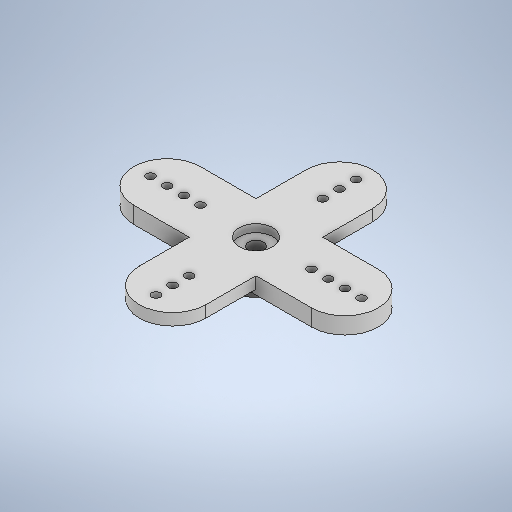
# Autodesk Inventor part: MMAE 232 Assignment 2_Servo Horn 3 - Dylan Tamras
Saved by Autodesk Inventor 2025.2 (Build 292293000, 293)
## iProperties
Created: 2025-01-19
Part Number: MMAE 232 Assignment 2_Servo Horn 3 - Dylan Tamras
Material: Generic
Document SubType Name: Modeling
Designer: Dylan
Density: 1 g/cm^3
Appearance: Default
Author: VRK99-0110
Title: Servo - Horn 3
Autodesk Inventor part; units mm, degrees
ref_plane "YZ Plane" through (0, 0, 0) normal (1, 0, 0) x (0, 1, 0)
ref_plane "XZ Plane" through (0, 0, 0) normal (0, 1, 0) x (-1, 0, 0)
ref_plane "XY Plane" through (0, 0, 0) normal (0, 0, 1) x (1, 0, 0)
sketch "Sketch1" plane through (0, 0, 0) normal (0, 1, 0) x (-1, 0, 0)
  line L0 (6, -15) -> (6, -6)
  line L1 (16, -6) -> (16, 0)
  line L2 (6, -15) -> (0, -15)
  line L3 (16, -6) -> (6, -6)
  arc A0 (0, -21) -> (6, -15) centre (0, -15) ccw
  arc A1 (16, -6) -> (22, 0) centre (16, 0) ccw
  line L4 (6, 15) -> (6, 6)
  line L5 (16, 6) -> (16, 0)
  line L6 (6, 15) -> (0, 15)
  line L7 (16, 6) -> (6, 6)
  arc A2 (6, 15) -> (0, 21) centre (0, 15) ccw
  arc A3 (22, 0) -> (16, 6) centre (16, 0) ccw
  line L8 (-6, -15) -> (-6, -6)
  line L9 (-16, -6) -> (-16, 0)
  line L10 (-6, -15) -> (0, -15)
  line L11 (-16, -6) -> (-6, -6)
  arc A4 (-6, -15) -> (0, -21) centre (0, -15) ccw
  arc A5 (-22, 0) -> (-16, -6) centre (-16, 0) ccw
  line L12 (-16, 6) -> (-16, 0)
  arc A6 (-16, 6) -> (-22, 0) centre (-16, 0) ccw
  line L13 (-16, 6) -> (-6, 6)
  line L14 (-6, 15) -> (-6, 6)
  line L15 (-6, 15) -> (0, 15)
  arc A7 (0, 21) -> (-6, 15) centre (0, 15) ccw
  point P0 (0, 0)
  dimension "d0" = 16
  dimension "d1" = 15
  constraints: 32 end point, 16 point on circle, 8 centre point, 8 coincident, 1 perpendicular, 1 vertical
  measures "d0" distance of point (0, 0) L1.end
  measures "d1" distance of point (0, 0) L2.end
extrude "Extrusion1" add sketch "Sketch1" along normal blind 2.85
sketch "Sketch2" plane through (0, 0, 0) normal (0, -1, 0) x (1, 0, 0)
  line L0 (-6, -15) -> (-6, -6) projected
  line L1 (-6, -6) -> (-6, -15)
  line L2 (6, -6) -> (6, -15) projected
  line L3 (6, -6) -> (6, -15)
  arc A0 (-6, -15) -> (6, -15) centre (0, -15) ccw
  line L4 (-6, -6) -> (6, -6)
  line L5 (-6, 15) -> (-6, 6)
  line L6 (6, 6) -> (6, 15)
  arc A1 (6, 15) -> (-6, 15) centre (0, 15) ccw
  line L7 (-6, 6) -> (6, 6)
  point P0 (0, 0)
  constraints: 12 end point, 4 point on circle, 2 centre point, 2 tangent, 2 vertical
extrude "Extrusion2" cut sketch "Sketch2" against normal blind 1.45
sketch "Sketch3" plane through (0, 2.85, 0) normal (0, 1, 0) x (1, 0, 0)
  circle A0 centre (16, 0) radius 0.75
  circle A1 centre (0, -15) radius 0.75
  circle A2 centre (10, 0) radius 0.75
  circle A3 centre (13, 0) radius 0.75
  circle A4 centre (19, 0) radius 0.75
  arc A5 (6, 15) -> (-6, 15) centre (0, 15) ccw projected
  arc A6 (-6, -15) -> (6, -15) centre (0, -15) ccw projected
  circle A7 centre (-16, 0) radius 0.75
  circle A8 centre (-10, 0) radius 0.75
  circle A9 centre (-13, 0) radius 0.75
  circle A10 centre (-19, 0) radius 0.75
  circle A11 centre (0, -12) radius 0.75
  circle A12 centre (0, -18) radius 0.75
  arc A13 (16, -6) -> (16, 6) centre (16, 0) ccw projected
  arc A14 (-16, 6) -> (-16, -6) centre (-16, 0) ccw projected
  circle A15 centre (0, 15) radius 0.75
  circle A16 centre (0, 12) radius 0.75
  circle A17 centre (0, 18) radius 0.75
  point P0 (0, 0)
  dimension "d10" = 1.5
  dimension "d12" = 1.5
  dimension "d14" = 1.5
  dimension "d17" = 1.5
  dimension "d19" = 1.5
  dimension "d22" = 1.5
  constraints: 14 centre point
  measures "d10" diameter of A1
  measures "d12" diameter of A2
  measures "d14" diameter of A3
  measures "d17" diameter of A4
  measures "d19" diameter of A11
  measures "d22" diameter of A12
extrude "Extrusion3" cut sketch "Sketch3" against normal blind 2.85
sketch "Sketch4" plane through (0, 2.85, 0) normal (0, 1, 0) x (1, 0, 0)
  circle A0 centre (0, 0) radius 3
  dimension "d25" = 6
  constraints: 1 centre point, 1 coincident
  measures "d25" diameter of A0
extrude "Extrusion4" cut sketch "Sketch4" against normal blind 1.4
sketch "Sketch5" plane through (0, 1.45, 0) normal (0, 1, 0) x (1, 0, 0)
  circle A0 centre (0, 0) radius 1.35
  dimension "d28" = 2.7
  constraints: 1 centre point, 1 coincident
  measures "d28" diameter of A0
extrude "Extrusion5" cut sketch "Sketch5" against normal blind 1.45
sketch "Sketch6" plane through (0, 1.45, 0) normal (0, -1, 0) x (1, 0, 0)
  circle A0 centre (0, 18) radius 0.75 projected
  circle A1 centre (0, 12) radius 0.75 projected
  circle A2 centre (0, 15) radius 0.75 projected
  line L0 (6, 6) -> (-6, 6) projected
  line L1 (6, 15) -> (6, 6) projected
  arc A3 (6, 15) -> (-6, 15) centre (0, 15) ccw projected
  line L2 (-6, 6) -> (-6, 15) projected
  point P0 (0, 0)
extrude "Extrusion6" add sketch "Sketch6" along normal blind 0.7
sketch "Sketch7" plane through (0, 1.45, 0) normal (0, -1, 0) x (1, 0, 0)
  circle A0 centre (0, -18) radius 0.75 projected
  circle A1 centre (0, -15) radius 0.75 projected
  circle A2 centre (0, -12) radius 0.75 projected
  line L0 (6, -6) -> (6, -15) projected
  line L1 (-6, -6) -> (6, -6) projected
  line L2 (-6, -15) -> (-6, -6) projected
  arc A3 (-6, -15) -> (6, -15) centre (0, -15) ccw projected
  point P0 (0, 0)
extrude "Extrusion7" add sketch "Sketch7" along normal blind 0.7
sketch "Sketch8" plane through (0, 0, 0) normal (0, -1, 0) x (1, 0, 0)
  circle A0 centre (0, 0) radius 1.35 projected
  circle A1 centre (13, 0) radius 0.75 projected
  circle A2 centre (-19, 0) radius 0.75 projected
  circle A3 centre (-16, 0) radius 0.75 projected
  circle A4 centre (16, 0) radius 0.75 projected
  circle A5 centre (10, 0) radius 0.75 projected
  circle A6 centre (-10, 0) radius 0.75 projected
  circle A7 centre (-13, 0) radius 0.75 projected
  circle A8 centre (19, 0) radius 0.75 projected
  line L0 (-16, 6) -> (16, 6) projected
  arc A9 (-16, 6) -> (-16, -6) centre (-16, 0) ccw projected
  line L1 (16, -6) -> (-16, -6) projected
  arc A10 (16, -6) -> (16, 6) centre (16, 0) ccw projected
extrude "Extrusion8" add sketch "Sketch8" along normal blind 0.15
sketch "Sketch9" plane through (0, -0.15, 0) normal (0, -1, 0) x (1, 0, 0)
  circle A0 centre (0, 0) radius 5
  dimension "d37" = 10
  constraints: 1 centre point, 1 coincident
  measures "d37" diameter of A0
extrude "Extrusion9" add sketch "Sketch9" along normal blind 2.85
sketch "Sketch10" plane through (0, -3, 0) normal (0, -1, 0) x (1, 0, 0)
  circle A0 centre (0, 0) radius 2.75
  dimension "d40" = 5.5
  constraints: 1 centre point, 1 coincident
  measures "d40" diameter of A0
extrude "Extrusion10" cut sketch "Sketch10" against normal blind 2.85
body "Solid1"
